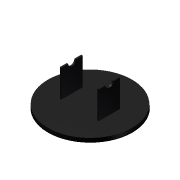
# Autodesk Inventor part: Shoulder
Saved by Autodesk Inventor 2012 (Build 160160000, 160)
## iProperties
Created: 2013-02-21
Part Number: Shoulder
Material: Default
Document SubType Name: Modeling
Designer: Andrew
Density: 1 g/cm^3
Author: Andrew
Autodesk Inventor part; units mm, degrees
ref_plane "YZ Plane" through (0, 0, 0) normal (1, 0, 0) x (0, 1, 0)
ref_plane "XZ Plane" through (0, 0, 0) normal (0, 1, 0) x (-1, 0, 0)
ref_plane "XY Plane" through (0, 0, 0) normal (0, 0, 1) x (1, 0, 0)
sketch "Sketch1" plane through (0, 0, 0) normal (0, 0, 1) x (1, 0, 0)
  circle A0 centre (0, 0) radius 55
  line L0 (23.5, -14) -> (23.5, 14)
  line L1 (-23.5, -14) -> (-23.5, 14)
  line L2 (-25.5, -14) -> (-25.5, 14)
  line L3 (25.5, -14) -> (25.5, 14)
  line L4 (25.5, 14) -> (23.5, 14)
  line L5 (23.5, -14) -> (25.5, -14)
  line L6 (-25.5, -14) -> (-23.5, -14)
  line L7 (-25.5, 14) -> (-23.5, 14)
  constraints: 8 end point, 3 equal length, 1 perpendicular
extrude "Extrusion1" add sketch "Sketch1" along normal blind 4.7625
extrude "Extrusion2" add sketch "Sketch1" along normal blind 40.7625 contours L0 L4 L3 L5 | L6 L2 L7 L1
sketch "Sketch2" plane through (25.5, -14, 4.7625) normal (1, 0, 0) x (0, 0, -1)
  line L0 (-36, 28) -> (-36, 0) projected
  line L1 (-39, 7) -> (-39, 2.0417)
  arc A0 (-39, 2.0417) -> (-37.1667, 0.0487) centre (-37, 2.0417) ccw
  arc A1 (-37.1667, 0.0487) -> (-36, 0) centre (-36, 14) ccw
  line L2 (-2, 0) -> (-36, 0)
  line L3 (-2, 28) -> (-2, 0)
  line L4 (-2, 28) -> (-36, 28)
  arc A2 (-36, 28) -> (-37.1667, 27.9513) centre (-36, 14) ccw
  arc A3 (-37.1667, 27.9513) -> (-39, 25.9583) centre (-37, 25.9583) ccw
  line L5 (-39, 25.9583) -> (-39, 21)
  arc A4 (-39, 21) -> (-37, 19) centre (-37, 21) ccw
  line L6 (-37, 19) -> (-36, 19)
  arc A5 (-36, 9) -> (-36, 19) centre (-36, 14) ccw
  line L7 (-37, 9) -> (-36, 9)
  arc A6 (-37, 9) -> (-39, 7) centre (-37, 7) ccw
  circle A7 centre (-36, 25) radius 1.25
  circle A8 centre (-28.2218, 21.7782) radius 1.25
  circle A9 centre (-25, 14) radius 1.25
  circle A10 centre (-28.2218, 6.2218) radius 1.25
  circle A11 centre (-36, 3) radius 1.25
  circle A12 centre (-15, 6) radius 1.05
  circle A13 centre (-15, 22) radius 1.05
  line L8 (-8, 6) -> (-11, 6)
  arc A14 (-12, 7) -> (-11, 6) centre (-11, 7) ccw
  line L9 (-12, 7) -> (-12, 21)
  arc A15 (-11, 22) -> (-12, 21) centre (-11, 21) ccw
  line L10 (-8, 22) -> (-11, 22)
  arc A16 (-7, 21) -> (-8, 22) centre (-8, 21) ccw
  line L11 (-7, 21) -> (-7, 7)
  arc A17 (-8, 6) -> (-7, 7) centre (-8, 7) ccw
  line L12 (-18, 21) -> (-18, 7)
  arc A18 (-19, 6) -> (-18, 7) centre (-19, 7) ccw
  line L13 (-19, 6) -> (-21, 6)
  arc A19 (-22, 7) -> (-21, 6) centre (-21, 7) ccw
  line L14 (-22, 7) -> (-22, 21)
  arc A20 (-21, 22) -> (-22, 21) centre (-21, 21) ccw
  line L15 (-21, 22) -> (-19, 22)
  arc A21 (-18, 21) -> (-19, 22) centre (-19, 21) ccw
  circle A22 centre (-36, 6) radius 1
  circle A23 centre (-28, 14) radius 1
  circle A24 centre (-36, 22) radius 1
  line L16 (-36, 19) -> (-36, 9)
  point P0 (4.7625, 14)
  point P1 (-36, 14)
  constraints: 32 end point, 30 point on circle, 25 centre point, 1 collinear, 1 midpoint
extrude "Extrusion3" cut sketch "Sketch2" against normal through all contours A5 L0
body "Solid1"
